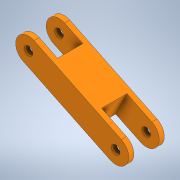
# Autodesk Inventor part: SECOND ARM
Saved by Autodesk Inventor 2021 (Build 250183000, 183)
## iProperties
Created: 2021-07-24
Part Number: SECOND ARM
Material: Generic
Document SubType Name: Modeling
Designer: aksha
Density: 1 g/cm^3
Appearance: Default
Author: aksha
Autodesk Inventor part; units mm, degrees
ref_plane "YZ Plane" through (0, 0, 0) normal (1, 0, 0) x (0, 1, 0)
ref_plane "XZ Plane" through (0, 0, 0) normal (0, 1, 0) x (-1, 0, 0)
ref_plane "XY Plane" through (0, 0, 0) normal (0, 0, 1) x (1, 0, 0)
sketch "Sketch1" plane through (0, 0, 0) normal (0, 0, 1) x (1, 0, 0)
  arc A0 (-32.5521, -67.5675) -> (32.5521, 67.5675) centre (0, 0) ccw
  circle A1 centre (0, 0) radius 25
  arc A2 (-473.7534, 311.4911) -> (-538.8576, 176.3561) centre (-506.3055, 243.9236) ccw
  circle A3 centre (-506.3055, 243.9236) radius 25
  line L0 (-473.7534, 311.4911) -> (32.5521, 67.5675)
  line L1 (-538.8576, 176.3561) -> (-32.5521, -67.5675)
  dimension "d0" = 150
  dimension "d1" = 50
  dimension "d2" = 150
  dimension "d3" = 50
  dimension "d4" = 562
  constraints: 4 centre point, 4 end point, 4 point on circle, 4 tangent, 3 coincident
  measures "d0" diameter of A0
  measures "d1" diameter of A1
  measures "d2" diameter of A2
  measures "d3" diameter of A3
  measures "d4" distance of L0.start L0.end
extrude "Extrusion1" add sketch "Sketch1" along normal blind 207
sketch "Sketch2" plane through (-473.7534, 311.4911, 207) normal (0.4340278, 0.9008995, 0) x (0.9008995, -0.4340278, 0)
  line L0 (116.8603, 30) -> (-116.8603, 30)
  line L1 (-116.8603, 30) -> (-116.8603, 177)
  line L2 (-116.8603, 177) -> (116.8603, 177)
  line L3 (116.8603, 177) -> (116.8603, 30)
  line L4 (0, 207) -> (0, 0) projected
  line L5 (116.8603, 30) -> (-116.8603, 177) construction
  line L6 (-116.8603, 30) -> (116.8603, 177) construction
  line L7 (-75, 0) -> (0, 0) projected
  point P0 (562, 207)
  point P1 (0, 103.5)
  dimension "d7" = 30
  constraints: 12 end point, 3 midpoint, 2 parallel, 1 horizontal, 1 perpendicular
  measures "d7" distance between parallel lines of L7 L0
extrude "Extrusion2" cut sketch "Sketch2" against normal blind 207
sketch "Sketch3" plane through (32.5521, 67.5675, 207) normal (0.4340278, 0.9008995, 0) x (0.9008995, -0.4340278, 0)
  line L0 (110.57, 177) -> (-160.57, 177)
  line L1 (-160.57, 177) -> (-160.57, 30)
  line L2 (-160.57, 30) -> (110.57, 30)
  line L3 (110.57, 30) -> (110.57, 177)
  line L4 (-25, 0) -> (-25, 207) projected
  line L5 (110.57, 177) -> (-160.57, 30) construction
  line L6 (-160.57, 177) -> (110.57, 30) construction
  point P0 (0, 207)
  point P1 (-25, 103.5)
  dimension "d10" = 30
  constraints: 12 end point, 3 midpoint, 2 parallel, 1 horizontal, 1 perpendicular
  measures "d10" distance from line of L4.end L0
extrude "Extrusion3" cut sketch "Sketch3" against normal blind 207
body "Solid1"
